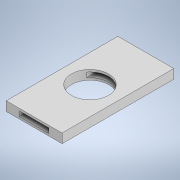
# Autodesk Inventor part: Peg toy top
Saved by Autodesk Inventor 2021 (Build 250183000, 183)
## iProperties
Created: 2020-12-18
Part Number: Peg toy top
Material: Generic
Document SubType Name: Modeling
Designer: Jawad
Density: 1 g/cm^3
Appearance: Default
Author: Jawad
Autodesk Inventor part; units mm, degrees
ref_plane "YZ Plane" through (0, 0, 0) normal (1, 0, 0) x (0, 1, 0)
ref_plane "XZ Plane" through (0, 0, 0) normal (0, 1, 0) x (-1, 0, 0)
ref_plane "XY Plane" through (0, 0, 0) normal (0, 0, 1) x (1, 0, 0)
sketch "Sketch1" plane through (0, 0, 0) normal (0, 1, 0) x (-1, 0, 0)
  line L0 (40.7614, 52.7865) -> (-35.4386, 52.7865)
  line L1 (-35.4386, 52.7865) -> (-35.4386, -99.6135)
  line L2 (-35.4386, -99.6135) -> (40.7614, -99.6135)
  line L3 (40.7614, -99.6135) -> (40.7614, 52.7865)
  circle A0 centre (2.6614, -23.4135) radius 25.4
  point P0 (0, 0)
  dimension "d0" = 152.4
  dimension "d1" = 76.2
  dimension "d2" = 50.8
  dimension "d5" = 76.2
  dimension "d6" = 38.1
  constraints: 8 end point, 2 parallel, 1 centre point, 1 horizontal, 1 perpendicular
  measures "d0" distance of L2.end L0.start
  measures "d1" distance of L1.end L2.end
  measures "d2" diameter of A0
  measures "d5" distance from line of L0 A0.centre
  measures "d6" distance from line of L3 A0.centre
extrude "Extrusion1" add sketch "Sketch1" along normal blind 12.7
sketch "Sketch2" plane through (-40.7614, 0, 52.7865) normal (0, 0, 1) x (1, 0, 0)
  line L0 (18.073, 9.7491) -> (58.127, 9.7491)
  line L1 (58.127, 9.7491) -> (58.127, 2.9509)
  line L2 (58.127, 2.9509) -> (18.073, 2.9509)
  line L3 (18.073, 2.9509) -> (18.073, 9.7491)
  line L4 (0, 12.7) -> (76.2, 12.7) projected
  line L5 (76.2, 0) -> (76.2, 12.7) projected
  line L6 (0, 0) -> (76.2, 0) projected
  line L7 (0, 0) -> (0, 12.7) projected
  point P0 (40.7614, 0)
  dimension "d9" = 2.9509
  dimension "d10" = 18.073
  dimension "d12" = 2.9509
  dimension "d13" = 18.073
  constraints: 8 end point, 2 parallel, 1 horizontal, 1 perpendicular
  measures "d9" distance between parallel lines of L4 L0
  measures "d10" distance between parallel lines of L5 L1
  measures "d12" distance from line of L6 L2.end
  measures "d13" distance between parallel lines of L7 L3
extrude "Extrusion2" cut sketch "Sketch2" against normal up to surface (152.4 mm away) contours L0 L1 L2 L3
equation "\"d1\" = 0.5 * d0"
equation "\"d5\" = 0.5 * d0"
equation "\"d6\" = 0.5 * d1"
equation "\"d12\" = d9"
equation "\"d13\" = d10"
body "Solid1"
